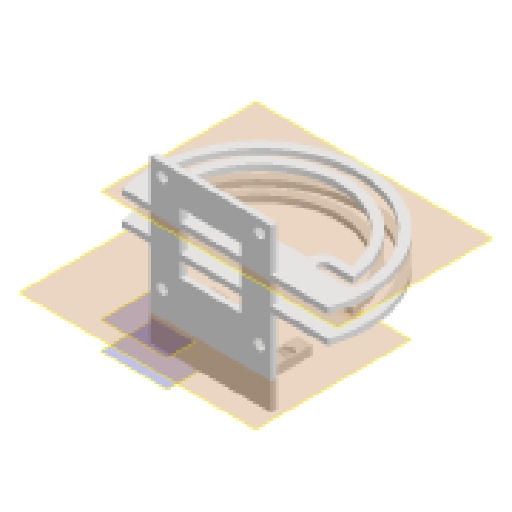
# Autodesk Inventor part: SG90_holder_1205
Saved by Autodesk Inventor 2024 (Build 280153000, 153)
## iProperties
Created: 2023-02-14
Part Number: SG90_holder_1205
Material: 一般
Document SubType Name: Modeling
Designer: USER
Density: 1 g/cm^3
Appearance: 預設
Author: USER
Autodesk Inventor part; units mm, degrees
ref_plane "YZ Plane" through (0, 0, 0) normal (1, 0, 0) x (0, 1, 0)
ref_plane "XY Plane" through (0, 0, 0) normal (0, 0, 1) x (1, 0, 0)
sketch "草圖22" plane through (0, 0, 0) normal (0, 0, 1) x (1, 0, 0)
  line L0 (-20, 20) -> (20, 20)
  line L1 (20, 20) -> (20, -20)
  line L2 (20, -20) -> (-20, -20)
  line L3 (-20, -20) -> (-20, 20)
  line L4 (0, -12.2) -> (0, 0) projected
  line L5 (-20, 20) -> (20, -20) construction
  line L6 (20, 20) -> (-20, -20) construction
  line L7 (-16, 16) -> (16, 16) construction
  line L8 (16, 16) -> (16, -16) construction
  line L9 (16, -16) -> (-16, -16) construction
  line L10 (-16, -16) -> (-16, 16) construction
  line L11 (-16, 16) -> (16, -16) construction
  line L12 (16, 16) -> (-16, -16) construction
  circle A0 centre (-16, 16) radius 1.65
  line L13 (20, 20) -> (-10, 20)
  line L14 (-10, 20) -> (-10, -10)
  line L15 (-10, -10) -> (20, -10)
  line L16 (20, -10) -> (20, 20)
  circle A1 centre (-16, -16) radius 1.65
  circle A2 centre (16, 16) radius 1.65
  circle A3 centre (16, -16) radius 1.65
  line L17 (-10, 10) -> (10, 10)
  line L18 (10, 10) -> (10, -10)
  line L19 (10, -10) -> (-10, -10)
  line L20 (-10, -10) -> (-10, 10)
  line L21 (-20, -20) -> (20, -20)
  line L22 (20, -20) -> (20, -33.437)
  line L23 (20, -33.437) -> (-20, -33.437)
  line L24 (-20, -33.437) -> (-20, -20)
  point P0 (20, -10)
  point P1 (10, -10)
  point P2 (-10, 10)
  dimension "d118" = 40
  dimension "d119" = 16
  dimension "d120" = 3.3
  dimension "d121" = 10
  dimension "d124" = 32
  dimension "d127" = 32
  constraints: 48 end point, 10 parallel, 6 perpendicular, 5 horizontal, 4 centre point, 4 midpoint, 2 collinear, 2 point on line, 1 coincident, 1 vertical, 9 other
  measures "d118" distance of L0.start L0.end
  measures "d119" distance from line of L4.end L8
  measures "d120" diameter of A0
  measures "d121" distance between parallel lines of L2 L15
  measures "d124" distance of A0.centre A1.centre
  measures "d127" distance of A0.centre A2.centre
extrude "擠出19" add sketch "草圖22" along normal blind 2 contours L0 L14 L15 L1 L2 L3 | L0 L1 L15 L18 L17 L14
ref_plane "工作平面5" through (0, -6, 0) normal (0, 1, 0) x (-1, 0, 0)
sketch "草圖31" plane through (0, 0, 0) normal (0, 1, 0) x (-1, 0, 0)
  line L0 (-16.35, 0) -> (16.35, 0)
  line L1 (16.35, 0) -> (16.35, -3)
  line L2 (16.35, -3) -> (-16.35, -3)
  line L3 (-16.35, -3) -> (-16.35, 0)
  line L4 (-16.35, 0) -> (16.35, -3) construction
  line L5 (16.35, 0) -> (-16.35, -3) construction
  line L6 (11.35, -3) -> (16.35, -3)
  line L7 (16.35, -3) -> (16.35, -15.2)
  line L8 (16.35, -15.2) -> (11.35, -15.2)
  line L9 (11.35, -15.2) -> (11.35, -3)
  line L10 (11.35, -3) -> (16.35, -15.2) construction
  line L11 (16.35, -3) -> (11.35, -15.2) construction
  line L12 (-11.35, -3) -> (-16.35, -3)
  line L13 (-16.35, -3) -> (-16.35, -15.2)
  line L14 (-16.35, -15.2) -> (-11.35, -15.2)
  line L15 (-11.35, -15.2) -> (-11.35, -3)
  line L16 (-11.35, -3) -> (-16.35, -15.2) construction
  line L17 (-16.35, -3) -> (-11.35, -15.2) construction
  line L18 (0, 0) -> (0, 15.4222) construction
  line L19 (-20, 0) -> (20, 0) construction
  circle A0 centre (13.8, -9.1) radius 1.15
  circle A1 centre (-13.8, -9.1) radius 1.15
  point P0 (0, -1.5)
  point P1 (13.85, -9.1)
  point P2 (-13.85, -9.1)
  dimension "d197" = 12.2
  dimension "d198" = 22.7
  dimension "d199" = 5
  dimension "d200" = 3
  dimension "d201" = 2.3
  dimension "d202" = 13.8
  constraints: 38 end point, 7 collinear, 6 midpoint, 6 parallel, 3 horizontal, 3 perpendicular, 2 centre point, 1 point on line, 1 symmetric about line, 1 vertical, 1 other
  measures "d197" distance of L6.end L7.end
  measures "d198" distance between parallel lines of L15 L9
  measures "d199" distance of L7.end L8.end
  measures "d200" distance between parallel lines of L0 L2
  measures "d201" diameter of A0
  measures "d202" horizontal distance of point (0, -1.5) A0.centre
extrude "擠出28" add sketch "草圖31" against normal blind 3 from surface at -6
ref_plane "工作平面11" through (0, -9, 0) normal (0, 1, 0) x (-1, 0, 0)
sketch "草圖35" plane through (0, -9, 0) normal (0, 1, 0) x (-1, 0, 0)
  line L0 (-10, 0) -> (10, 0) projected
  line L1 (10, 0) -> (16.35, 0) projected
  line L2 (16.35, 0) -> (16.35, -15.2) projected
  line L3 (16.35, -15.2) -> (11.35, -15.2) projected
  line L4 (11.35, -15.2) -> (11.35, -3) projected
  line L5 (11.35, -3) -> (-11.35, -3) projected
  line L6 (-11.35, -3) -> (-11.35, -15.2) projected
  line L7 (-11.35, -15.2) -> (-16.35, -15.2) projected
  line L8 (-16.35, -15.2) -> (-16.35, 0) projected
  line L9 (-16.35, 0) -> (-10, 0) projected
  circle A0 centre (-13.8, -9.1) radius 1.15 projected
  circle A1 centre (13.8, -9.1) radius 1.15 projected
  line L10 (15.3464, -10.7636) -> (15.3464, -7.0453)
  line L11 (-12.2601, -11.0386) -> (-12.2601, -6.8072)
  line L12 (16.0139, -8.5926) -> (12.7938, -6.7335)
  line L13 (14.4675, -6.929) -> (11.2474, -8.7881)
  line L14 (12.2536, -7.4364) -> (12.2536, -11.1547)
  line L15 (11.5861, -9.6074) -> (14.8062, -11.4665)
  line L16 (13.1325, -11.271) -> (16.3526, -9.4119)
  line L17 (-11.3512, -8.7357) -> (-15.0157, -6.62)
  line L18 (-12.8911, -6.7972) -> (-16.5555, -8.9128)
  line L19 (-15.3399, -7.1614) -> (-15.3399, -11.3928)
  line L20 (-16.2488, -9.4643) -> (-12.5843, -11.58)
  line L21 (-14.7089, -11.4028) -> (-11.0445, -9.2872)
  point P0 (0, 0)
  point P1 (13.8, -10.8856)
  point P2 (15.3464, -9.9928)
  point P3 (15.3464, -8.2072)
  point P4 (13.8, -7.3144)
  point P5 (12.2536, -8.2072)
  point P6 (12.2536, -9.9928)
  point P7 (-13.8, -10.8781)
  point P8 (-12.2601, -9.989)
  point P9 (-12.2601, -8.211)
  point P10 (-13.8, -7.3219)
  point P11 (-15.3399, -8.211)
  point P12 (-15.3399, -9.989)
  dimension "d254" = 360
  dimension "d258" = 360
  constraints: 24 end point, 2 vertical, 38 other
extrude "擠出32" cut sketch "草圖35" along normal blind 2 contours L18 L17 L11 L21 L20 L19 | L16 L15 L14 L13 L12 L10
